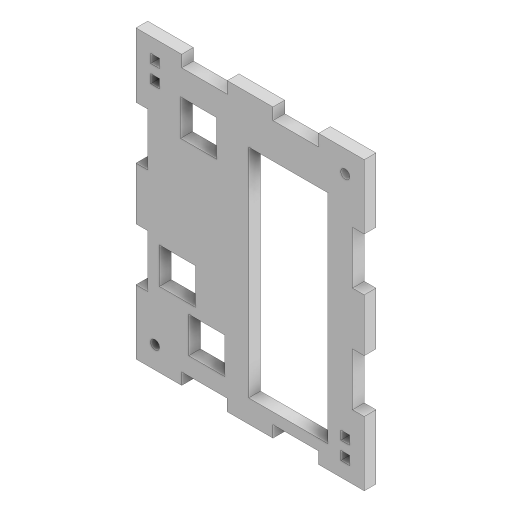
# Autodesk Inventor part: Top
Saved by Autodesk Inventor 2023.3 (Build 273359000, 359)
## iProperties
Created: 2024-06-25
Part Number: Top
Material: Generic
Document SubType Name: Modeling
Designer: David Zindović
Density: 1 g/cm^3
Appearance: Default
Author: David Zindović
Autodesk Inventor part; units mm, degrees
ref_plane "YZ Plane" through (0, 0, 0) normal (1, 0, 0) x (0, 1, 0)
ref_plane "XZ Plane" through (0, 0, 0) normal (0, 1, 0) x (-1, 0, 0)
ref_plane "XY Plane" through (0, 0, 0) normal (0, 0, 1) x (1, 0, 0)
sketch "Sketch1" plane through (0, 0, 0) normal (0, 0, 1) x (1, 0, 0)
  line L0 (-39, 49) -> (39, 49)
  line L1 (39, 49) -> (39, -49)
  line L2 (39, -49) -> (-39, -49)
  line L3 (-39, -49) -> (-39, 49)
  line L4 (-23.4, -45) -> (-7.8, -45)
  line L5 (-7.8, -45) -> (-7.8, -49)
  line L6 (-7.8, -49) -> (-23.4, -49)
  line L7 (-23.4, -49) -> (-23.4, -45)
  line L8 (-39, -27) -> (-35, -27)
  line L9 (-35, -27) -> (-35, -9)
  line L10 (-35, -9) -> (-39, -9)
  line L11 (-39, -9) -> (-39, -27)
  line L12 (0, 0) -> (8.9596, 0)
  line L13 (0, 0) -> (0, 8.0367)
  line L14 (-23.4, 45) -> (-7.8, 45)
  line L15 (-7.8, 45) -> (-7.8, 49)
  line L16 (-23.4, 49) -> (-23.4, 45)
  line L17 (-39, 27) -> (-35, 27)
  line L18 (-35, 27) -> (-35, 9)
  line L19 (-35, 9) -> (-39, 9)
  line L20 (23.4, -45) -> (7.8, -45)
  line L21 (7.8, -45) -> (7.8, -49)
  line L22 (23.4, -49) -> (23.4, -45)
  line L23 (39, -27) -> (35, -27)
  line L24 (35, -27) -> (35, -9)
  line L25 (35, -9) -> (39, -9)
  line L26 (0, 0) -> (-8.9596, 0)
  line L27 (39, 27) -> (35, 27)
  line L28 (35, 27) -> (35, 9)
  line L29 (35, 9) -> (39, 9)
  line L30 (7.8, 45) -> (7.8, 49)
  line L31 (23.4, 49) -> (23.4, 45)
  line L32 (23.4, 45) -> (7.8, 45)
  point P0 (0, 49)
  point P1 (39, 0)
  point P2 (0, -49)
  point P3 (-7.8, -47)
  point P4 (-37, -9)
  dimension "d0" = 98
  dimension "d1" = 78
  dimension "d2" = 15.6
  dimension "d3" = 4
  dimension "d4" = 4
  dimension "d5" = 18
  dimension "d6" = 7.8
  dimension "d7" = 9
  constraints: 66 end point, 25 symmetric about line, 6 parallel, 5 midpoint, 4 horizontal, 3 perpendicular, 2 collinear, 1 horizontal alignment, 1 vertical, 1 vertical alignment
  measures "d0" distance of L0.end L1.end
  measures "d1" distance of L0.start L0.end
  measures "d2" distance of L5.end L6.end
  measures "d3" distance of L4.end L5.end
  measures "d4" distance of L10.end L9.end
  measures "d5" distance of L9.end L8.end
  measures "d6" horizontal distance of point (0, -49) point (-7.8, -47)
  measures "d7" vertical distance of L12.start point (-37, -9)
extrude "Extrusion1" add sketch "Sketch1" along normal mid plane 4 contours L0 L16 L14 L15 L30 L32 L31 L1 L27 L28 L29 L25 L24 L23 L2 L22 L20 L21 L5 L4 L7 L3 L8 L9 L10 L19 L18 L17
sketch "Sketch2" plane through (0, 0, 2) normal (0, 0, 1) x (1, 0, 0)
  line L0 (-21, -39) -> (-8.7, -39)
  line L1 (-8.7, -39) -> (-8.7, -26.7)
  line L2 (-8.7, -26.7) -> (-21, -26.7)
  line L3 (-21, -26.7) -> (-21, -39)
  line L4 (-35, -9) -> (-35, -27) projected
  line L5 (-23.4, -45) -> (-7.8, -45) projected
  line L6 (-18.7, -11.2) -> (-31, -11.2)
  line L7 (-31, -11.2) -> (-31, -23.5)
  line L8 (-31, -23.5) -> (-18.7, -23.5)
  line L9 (-18.7, -23.5) -> (-18.7, -11.2)
  line L10 (-11.45, 36.25) -> (-23.75, 36.25)
  line L11 (-23.75, 36.25) -> (-23.75, 23.95)
  line L12 (-23.75, 23.95) -> (-11.45, 23.95)
  line L13 (-11.45, 23.95) -> (-11.45, 36.25)
  line L14 (-7.8, 45) -> (-23.4, 45) projected
  line L15 (-35, 27) -> (-35, 9) projected
  line L16 (26.6, 33) -> (-0.5, 33)
  line L17 (-0.5, 33) -> (-0.5, -41.25)
  line L18 (-0.5, -41.25) -> (26.6, -41.25)
  line L19 (26.6, -41.25) -> (26.6, 33)
  line L20 (23.4, 45) -> (7.8, 45) projected
  circle A0 centre (-32.5, -41.5) radius 1.55
  circle A1 centre (32.5, 41.5) radius 1.55
  line L21 (35, 9) -> (35, 27) projected
  line L22 (-31, 44) -> (-34, 44)
  line L23 (-34, 44) -> (-34, 41)
  line L24 (-34, 41) -> (-31, 41)
  line L25 (-31, 41) -> (-31, 44)
  line L26 (-34, 38) -> (-31, 38)
  line L27 (-31, 38) -> (-31, 35)
  line L28 (-31, 35) -> (-34, 35)
  line L29 (-34, 35) -> (-34, 38)
  line L30 (0, 0) -> (5.8135, 0)
  line L31 (0, 0) -> (0, 4.2513)
  line L32 (34, -35) -> (31, -35)
  line L33 (31, -35) -> (31, -38)
  line L34 (31, -38) -> (34, -38)
  line L35 (34, -38) -> (34, -35)
  line L36 (31, -41) -> (34, -41)
  line L37 (34, -41) -> (34, -44)
  line L38 (34, -44) -> (31, -44)
  line L39 (31, -44) -> (31, -41)
  line L40 (7.8, -45) -> (23.4, -45) projected
  line L41 (35, -27) -> (35, -9) projected
  point P0 (-17.6, 36.25)
  point P1 (-8.7, -32.85)
  dimension "d10" = 12.3
  dimension "d11" = 12.3
  dimension "d12" = 14
  dimension "d13" = 6
  dimension "d14" = 4
  dimension "d15" = 21.5
  dimension "d16" = 12.3
  dimension "d17" = 12.3
  dimension "d18" = 8.75
  dimension "d19" = 11.25
  dimension "d20" = 12.3
  dimension "d21" = 12.3
  dimension "d23" = 74.25
  dimension "d24" = 27.1
  dimension "d25" = 34.5
  dimension "d26" = 12
  dimension "d29" = 3.1
  dimension "d30" = 3.5
  dimension "d31" = 2.5
  dimension "d32" = 3.1
  dimension "d33" = 3.5
  dimension "d34" = 2.5
  dimension "d35" = 3
  dimension "d36" = 3
  dimension "d37" = 1
  dimension "d38" = 3
  dimension "d39" = 3
  dimension "d40" = 1
  dimension "d41" = 3
  dimension "d42" = 3
  dimension "d43" = 3
  dimension "d44" = 3
  dimension "d45" = 3
  dimension "d46" = 3
  dimension "d47" = 1
  dimension "d48" = 1
  constraints: 68 end point, 16 parallel, 9 horizontal, 8 perpendicular, 2 centre point, 2 midpoint, 2 vertical alignment, 1 vertical
  measures "d10" distance of L2.end L0.start
  measures "d11" distance of L0.start L0.end
  measures "d12" distance between parallel lines of L3 L4
  measures "d13" distance between parallel lines of L5 L0
  measures "d14" distance between parallel lines of L7 L4
  measures "d15" distance between parallel lines of L5 L8
  measures "d16" distance of L6.end L7.end
  measures "d17" distance of L7.end L8.end
  measures "d18" distance from line of L14 point (-17.6, 36.25)
  measures "d19" distance between parallel lines of L15 L11
  measures "d20" distance of L10.end L11.end
  measures "d21" distance of L11.end L12.end
  measures "d23" distance of L18.end L16.start
  measures "d24" distance of L17.end L18.end
  measures "d25" distance between parallel lines of L17 L15
  measures "d26" distance between parallel lines of L20 L16
  measures "d29" diameter of A0
  measures "d30" distance from line of L5 A0.centre
  measures "d31" distance from line of L4 A0.centre
  measures "d32" diameter of A1
  measures "d33" distance from line of L20 A1.centre
  measures "d34" distance from line of L21 A1.centre
  measures "d35" distance of L24.end L23.end
  measures "d36" distance of L23.end L22.end
  measures "d37" distance between parallel lines of L14 L22
  measures "d38" distance of L26.end L27.end
  measures "d39" distance of L27.end L28.end
  measures "d40" distance between parallel lines of L15 L29
  measures "d41" distance between parallel lines of L24 L26
  measures "d42" distance of L34.end L34.start
  measures "d43" distance of L34.start L33.start
  measures "d44" distance of L37.start L38.start
  measures "d45" distance of L38.start L38.end
  measures "d46" distance between parallel lines of L34 L36
  measures "d47" distance between parallel lines of L40 L38
  measures "d48" distance between parallel lines of L41 L35
extrude "Extrusion2" cut sketch "Sketch2" against normal up to surface (4 mm away)
equation "\"d6\" = 0.5 * d2"
equation "\"d7\" = 0.5 * d5"
equation "\"d11\" = d10"
equation "\"d16\" = d10"
equation "\"d17\" = d10"
equation "\"d20\" = d16"
equation "\"d21\" = d20"
equation "\"d32\" = d29"
equation "\"d33\" = d30"
equation "\"d34\" = d31"
equation "\"d36\" = d35"
equation "\"d38\" = d36"
equation "\"d39\" = d35"
equation "\"d43\" = d42"
equation "\"d44\" = d43"
equation "\"d45\" = d42"
equation "\"d47\" = d37"
equation "\"d48\" = d47"
body "Solid1"
